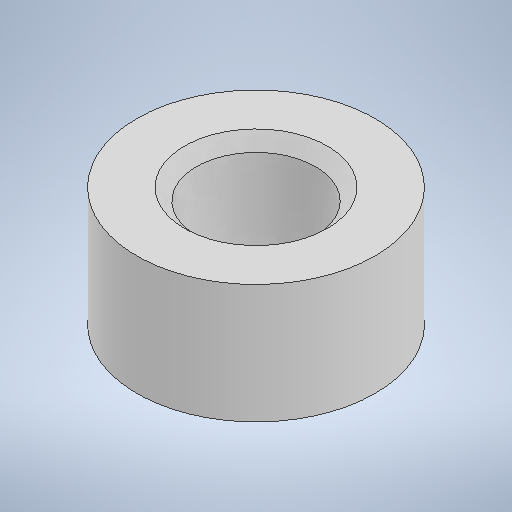
# Autodesk Inventor part: TS_Magazin_Gleitbuchse_int
Saved by Autodesk Inventor 2025.2 (Build 292293000, 293)
## iProperties
Created: 2025-06-01
Part Number: TS_Magazin_Gleitbuchse_int
Material: Generisch
Document SubType Name: Modeling
Designer: tino
Density: 1 g/cm^3
Appearance: Vorgabe
Author: tino
Autodesk Inventor part; units mm, degrees
ref_plane "YZ Plane" through (0, 0, 0) normal (1, 0, 0) x (0, 1, 0)
ref_plane "XZ Plane" through (0, 0, 0) normal (0, 1, 0) x (-1, 0, 0)
ref_plane "XY Plane" through (0, 0, 0) normal (0, 0, 1) x (1, 0, 0)
sketch "Skizze1" plane through (0, 0, 0) normal (0, 0, 1) x (1, 0, 0)
  circle A0 centre (0, 0) radius 10
  dimension "d0" = 20
  constraints: 1 centre point, 1 coincident
  measures "d0" diameter of A0
extrude "Extrusion1" add sketch "Skizze1" along normal mid plane 10
sketch "Skizze2" plane through (0, 0, 5) normal (0, 0, 1) x (1, 0, 0)
  point P0 (0, 0)
  point P1 (0, 0)
  constraints: 1 coincident
hole "Bohrung1" at (0, 0, 5) direction (0, 0, -1) diameter 10 end through all
chamfer "Fasen1" distance 1 angle 45 2 edges at (0, 5, 5) (0, 5, -5)
equation "\"d0\" = Gleitbuchse_Aussendurchmesser"
equation "\"d1\" = Hoehe_Buchse"
equation "\"d3\" = Gleitbuchse_Innendurchmesser"
equation "\"d10\" = Fase"
equation "\"Gleitbuchse_Aussendurchmesser\" = 20"
equation "\"Gleitbuchse_Innendurchmesser\" = 10"
equation "\"Hoehe_Buchse\" = 10"
equation "\"Fase\" = 1"
